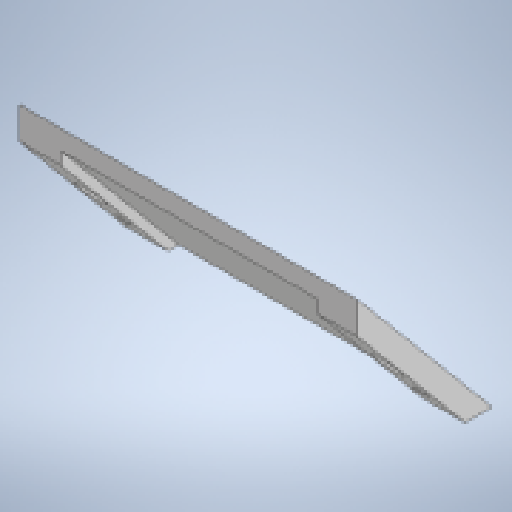
# Autodesk Inventor part: MS_Pokrywa
Saved by Autodesk Inventor 2023 (Build 270158000, 158)
## iProperties
Created: 2024-04-29
Part Number: MS_Pokrywa
Material: Ogólny
Document SubType Name: Modeling
Designer: kamil
Density: 1 g/cm^3
Appearance: Domyślna
Author: kamil
Autodesk Inventor part; units mm, degrees
ref_plane "YZ Plane" through (0, 0, 0) normal (1, 0, 0) x (0, 1, 0)
ref_plane "XZ Plane" through (0, 0, 0) normal (0, 1, 0) x (-1, 0, 0)
ref_plane "XY Plane" through (0, 0, 0) normal (0, 0, 1) x (1, 0, 0)
sketch "Szkic1" plane through (0, 0, 0) normal (1, 0, 0) x (0, 1, 0)
  line L0 (0, 0) -> (0, 3.916)
  line L1 (0, 3.916) -> (34.0032, 32.4481)
  line L2 (0, 0) -> (34.0032, 28.5321)
  line L3 (34.0032, 28.5321) -> (38.6701, 32.4481)
  line L4 (34.0032, 32.4481) -> (38.6701, 32.4481)
  dimension "d0" = 3.916
  dimension "d1" = 130
  dimension "d2" = 44.388
  constraints: 10 end point, 1 collinear, 1 horizontal, 1 horizontal alignment, 1 parallel, 1 vertical
  measures "d0" distance of L0.start L0.end
  measures "d1" angle of L0 L1
  measures "d2" distance of L0.end L1.end
extrude "Wyciągnięcie proste1" add sketch "Szkic1" against normal blind 82
sketch "Szkic2" plane through (0, 0, 0) normal (0, 0.6427876, -0.7660444) x (-1, 0, 0)
  circle A0 centre (5, 7.1954) radius 2.85 projected
  circle A1 centre (77, 7.1954) radius 2.85 projected
  point P0 (0, 0)
move faces "Przesuń1" translate (0, -1.2856, 1.5321) faces at (-27.3333, 22.6688, 22.9374)
sketch "Szkic3" plane through (-82, 30.8917, 32.4481) normal (0, -0.6427876, 0.7660444) x (1, 0, 0)
  line L0 (82, 5.9586) -> (82, 0) projected
  line L1 (82, 5.9586) -> (0, 5.9586) projected
  line L2 (0, 0) -> (0, 5.9586) projected
  line L3 (82, 0) -> (0, 0) projected
  line L4 (82, 0) -> (82, -40.3263) projected
  line L5 (82, 0) -> (0, 0) projected
  line L6 (0, -40.3263) -> (0, 0) projected
  line L7 (82, -40.3263) -> (0, -40.3263) projected
  line L8 (82, -40.3263) -> (82, -44.5216) projected
  line L9 (82, -40.3263) -> (0, -40.3263) projected
  line L10 (0, -44.5216) -> (0, -40.3263) projected
  line L11 (82, -44.5216) -> (0, -44.5216) projected
  line L12 (10, 5.9586) -> (72, 5.9586)
  line L13 (72, 5.9586) -> (72, -44.5216)
  line L14 (72, -44.5216) -> (10, -44.5216)
  line L15 (10, -44.5216) -> (10, 5.9586)
  point P0 (0, -20.1631)
  point P1 (10, -44.5216)
  point P2 (72, 5.9586)
  dimension "d9" = 10
  dimension "d10" = 10
  constraints: 8 end point, 2 parallel, 2 point on line, 1 horizontal, 1 midpoint, 1 perpendicular
  measures "d9" distance between parallel lines of L4 L13
  measures "d10" distance from line of L15 point (0, -20.163)
extrude "Wyciągnięcie proste2" cut sketch "Szkic3" against normal blind 2 contours L13 L3 L15 L1 | L13 L7 L15 L3 | L13 L11 L15 L7
hole "Otwór1" at (-5, 5.512, 4.6251) at (-77, 5.512, 4.6251) direction (0, -0.6427876, 0.7660444) diameter 3.2 depth 4.9998 counterbore diameter 5.7 counterbore depth 3.1
sketch "Szkic4" plane through (-82, 38.6701, 32.4481) normal (0, 0, 1) x (1, 0, 0)
  circle A0 centre (77, -21.1701) radius 3 projected
  circle A1 centre (5, -21.1701) radius 3 projected
  point P0 (82, -38.6701)
extrude "Wyciągnięcie proste3" cut sketch "Szkic4" against normal through all
